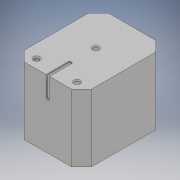
# Autodesk Inventor part: Kozhuh_Lock
Saved by Autodesk Inventor 2017 (Build 210142000, 142)
## iProperties
Part Number: Kozhuh_Lock
Material: Типовые
Document SubType Name: Modeling
Designer: yulia_000
Density: 1 g/cm^3
Appearance: По умолчанию
Author: yulia_000
## iProperties of the stored document Kozhuh_Lock_3DПЕЧАТЬ.ipt
Part Number: Kozhuh_Lock_3DПЕЧАТЬ
Material: Типовые
Document SubType Name: Modeling
Designer: yulia_000
Density: 1 g/cm^3
Appearance: По умолчанию
Author: yulia_000
Autodesk Inventor part; units mm, degrees
ref_plane "YZ Plane" through (0, 0, 0) normal (1, 0, 0) x (0, 1, 0)
ref_plane "XZ Plane" through (0, 0, 0) normal (0, 1, 0) x (-1, 0, 0)
ref_plane "XY Plane" through (0, 0, 0) normal (0, 0, 1) x (1, 0, 0)
sketch "Эскиз1" plane through (0, 0, 0) normal (0, 1, 0) x (-1, 0, 0)
  line L0 (8.5, 0) -> (50.1, 0)
  line L1 (58.6, -8.5) -> (58.6, -65.5)
  line L2 (50.1, -74) -> (8.5, -74)
  line L3 (0, -65.5) -> (0, -8.5)
  line L4 (58.6, -8.5) -> (50.1, 0)
  line L5 (58.6, -65.5) -> (50.1, -74)
  line L6 (8.5, -74) -> (0, -65.5)
  line L7 (0, -8.5) -> (8.5, 0)
  line L8 (59.8, -65.9971) -> (50.5971, -75.2)
  line L9 (50.5971, -75.2) -> (8.0029, -75.2)
  line L10 (8.0029, -75.2) -> (-1.2, -65.9971)
  line L11 (-1.2, -65.9971) -> (-1.2, -8.0029)
  line L12 (-1.2, -8.0029) -> (8.0029, 1.2)
  line L13 (8.0029, 1.2) -> (50.5971, 1.2)
  line L14 (50.5971, 1.2) -> (59.8, -8.0029)
  line L15 (59.8, -8.0029) -> (59.8, -65.9971)
  line L16 (30.8, -54) -> (27.8, -54)
  line L17 (27.8, -54) -> (27.8, -74)
  line L18 (27.8, -74) -> (30.8, -74)
  line L19 (30.8, -74) -> (30.8, -54)
  line L20 (30.8, -54) -> (27.8, -74) construction
  line L21 (27.8, -54) -> (30.8, -74) construction
  point P0 (0, 0)
  point P1 (58.6, -74)
  point P2 (58.6, 0)
  point P3 (0, -74)
  point P4 (29.3, -64)
  point P5 (29.3, -74)
  dimension "d8" = 58.6
  dimension "d9" = 74
  dimension "d10" = 8.5
  dimension "d11" = 8.5
  dimension "d12" = 8.5
  dimension "d13" = 8.5
  dimension "d14" = 8.5
  dimension "d15" = 8.5
  dimension "d16" = 8.5
  dimension "d17" = 8.5
  dimension "d18" = 1.2
  dimension "d51" = 3
  dimension "d52" = 20
  constraints: 44 end point, 8 point on line, 6 parallel, 4 midpoint, 3 perpendicular, 2 horizontal, 7 other
  measures "d8" distance of point (58.6, -74) point (0, -74)
  measures "d9" distance of point (58.6, 0) point (58.6, -74)
  measures "d10" distance of L1.start point (58.6, 0)
  measures "d11" distance of L0.end point (58.6, 0)
  measures "d12" distance of L1.end point (58.6, -74)
  measures "d13" distance of L2.start point (58.6, -74)
  measures "d14" distance of L2.end point (0, -74)
  measures "d15" distance of L3.start point (0, -74)
  measures "d16" distance of L3.end point (0, 0)
  measures "d17" distance of L0.start point (0, 0)
  measures "d18" distance between parallel lines of L1 L15
  measures "d51" distance of L18.end L17.end
  measures "d52" distance of L17.end L16.end
extrude "Выдавливание1" add sketch "Эскиз1" against normal blind 1 contours L0 L4 L1 L5 L2 L19 L16 L17 L6 L3 L7 | L17 L16 L19 L2 | L8 L9 L10 L11 L12 L13 L14 L15
extrude "Выдавливание2" add sketch "Эскиз1" along normal blind 60
fillet "Сопряжение1" radius 1 8 edges at (-58.6, 0, -37) (-54.35, 0, -69.75) (-29.3, 0, -74) (-4.25, 0, -69.75) (0, 0, -37) (-4.25, 0, -4.25) (-29.3, 0, 0) (-54.35, 0, -4.25)
extrude "Выдавливание3" add sketch "Эскиз1" along normal blind 18 separate body contours L17 L16 L19 L2
sketch "Эскиз2" plane through (-27.8, 0, -74) normal (0, 0, -1) x (-1, 0, 0)
  line L0 (0, 0) -> (3, 0) projected
  line L1 (3, 0) -> (3, 18) projected
  line L2 (0, 18) -> (3, 18) projected
  line L3 (0, 0) -> (0, 18) projected
  point P0 (-27.8, 0)
extrude "Выдавливание4" add sketch "Эскиз2" along normal blind 18 bodies 2
sketch "Эскиз3" plane through (0, 0, 0) normal (0, -1, 0) x (1, 0, 0)
  line L0 (-27.8, -54) -> (-27.8, -92) projected
  line L1 (-30.8, -54) -> (-27.8, -54) projected
  line L2 (-30.8, -54) -> (-30.8, -92) projected
  line L3 (-27.8, -92) -> (-30.8, -92) projected
  point P0 (0, 0)
extrude "Выдавливание5" add sketch "Эскиз3" along normal blind 18 bodies 2
combine bodies "Комбинировать1" operation type subtract main body 1 bodies to subtract 2
hole "Отверстие4" at (-47.6, -1, -67) direction (0, 1, 0) diameter 4.2 end through all countersink diameter 6 countersink angle 90 bodies 1
hole "Отверстие5" at (-11, -1, -67) direction (0, 1, 0) diameter 4.2 end through all countersink diameter 6 countersink angle 90 bodies 1
hole "Отверстие6" at (-29, -1, -32) direction (0, 1, 0) diameter 4.2 end through all countersink diameter 6 countersink angle 90 bodies 1
fillet "Сопряжение2" radius 1 16 edges at (-58.3071, 0.2929, -65.3787) (-58.6, 30.5, -65.5) (-49.9787, 0.2929, -73.7071) (-50.1, 30.5, -74) (-8.6213, 0.2929, -73.7071) (-8.5, 30.5, -74) (-0.2929, 0.2929, -65.3787) (0, 30.5, -65.5) (-0.2929, 0.2929, -8.6213) (0, 30.5, -8.5) (-8.6213, 0.2929, -0.2929) (-8.5, 30.5, 0) (-49.9787, 0.2929, -0.2929) (-50.1, 30.5, 0) (-58.3071, 0.2929, -8.6213) (-58.6, 30.5, -8.5)
fillet "Сопряжение3" radius 1 4 edges at (-30.8, -0.5, -54) (-27.8, -0.5, -54) (-27.8, 18, -74.6) (-30.8, 18, -74.6)
equation "\"d11\" = d10"
equation "\"d12\" = d10"
equation "\"d13\" = d12"
equation "\"d14\" = d10"
equation "\"d15\" = d14"
equation "\"d16\" = d10"
equation "\"d17\" = d16"
